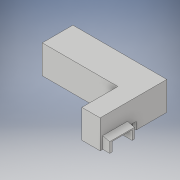
# Autodesk Inventor part: Батарейка
Saved by Autodesk Inventor 2019 (Build 230136000, 136)
## iProperties
Created: 2018-06-26
Part Number: Батарейка
Material: Типовые
Document SubType Name: Modeling
Designer: rossolov
Density: 1 g/cm^3
Appearance: По умолчанию
Author: rossolov
Autodesk Inventor part; units mm, degrees
ref_plane "YZ Plane" through (0, 0, 0) normal (1, 0, 0) x (0, 1, 0)
ref_plane "XZ Plane" through (0, 0, 0) normal (0, 1, 0) x (-1, 0, 0)
ref_plane "XY Plane" through (0, 0, 0) normal (0, 0, 1) x (1, 0, 0)
sketch "Эскиз1" plane through (0, 0, 0) normal (0, 0, 1) x (1, 0, 0)
  line L0 (-41.9106, 11.3854) -> (9.5324, 11.3854)
  line L1 (9.5324, 11.3854) -> (9.5324, -4.2346)
  line L2 (9.5324, -4.2346) -> (-41.9106, -4.2346)
  line L3 (-41.9106, -4.2346) -> (-41.9106, 11.3854)
  point P0 (0, 0)
  dimension "d0" = 51.443
  dimension "d1" = 15.62
  constraints: 8 end point, 2 parallel, 1 horizontal, 1 perpendicular
  measures "d0" distance of L1.end L2.end
  measures "d1" distance of L0.end L1.end
extrude "Выдавливание1" add sketch "Эскиз1" against normal blind 16.769
sketch "Эскиз2" plane through (9.5324, -4.2346, 0) normal (1, 0, 0) x (0, 0, -1)
  line L0 (0, 15.62) -> (16.769, 15.62) projected
  line L1 (16.769, 15.62) -> (-19.74, 15.62)
  line L2 (-19.74, 15.62) -> (-19.74, 0)
  line L3 (-19.74, 0) -> (16.769, 0)
  line L4 (16.769, 0) -> (16.769, 15.62)
  point P0 (0, 4.2346)
  dimension "d4" = 36.509
  constraints: 8 end point, 2 parallel, 1 horizontal, 1 perpendicular
  measures "d4" distance of L3.end L2.end
extrude "Выдавливание2" add sketch "Эскиз2" against normal blind 10
sketch "Эскиз3" plane through (9.5324, -4.2346, -16.769) normal (1, 0, 0) x (0, 0, -1)
  line L0 (0, 15.62) -> (0, 0) projected
  line L1 (-36.509, 0) -> (0, 0) projected
  line L2 (-16.769, 0) -> (-21.568, 0)
  line L3 (-21.568, 0) -> (-21.568, 4.078)
  line L4 (-21.568, 4.078) -> (-16.769, 4.078)
  line L5 (-16.769, 4.078) -> (-16.769, 0)
  point P0 (-16.769, 4.2346)
  dimension "d7" = 16.769
  dimension "d8" = 4.799
  dimension "d9" = 4.078
  constraints: 8 end point, 2 parallel, 1 horizontal, 1 perpendicular, 1 point on line
  measures "d7" distance of L0.end L2.start
  measures "d8" distance of L3.end L4.end
  measures "d9" distance of L2.end L3.end
extrude "Выдавливание3" cut sketch "Эскиз3" against normal blind 1.867
sketch "Эскиз4" plane through (-0.4676, -4.2346, 0) normal (-1, 0, 0) x (0, 0, 1)
  line L0 (19.74, 15.62) -> (19.74, 0) projected
  line L1 (18.24, 1.5) -> (1.5, 1.5)
  line L2 (1.5, 1.5) -> (1.5, 14.12)
  line L3 (1.5, 14.12) -> (18.24, 14.12)
  line L4 (18.24, 14.12) -> (18.24, 1.5)
  point P0 (0, 4.2346)
  constraints: 8 end point, 2 parallel, 1 horizontal, 1 perpendicular
extrude "Выдавливание4" cut sketch "Эскиз4" against normal blind 7.5
sketch "Эскиз6" plane through (9.5324, -4.2346, -16.769) normal (1, 0, 0) x (0, 0, -1)
  line L0 (-16.769, 0) -> (-36.509, 0) projected
  line L1 (-21.817, 0) -> (-22.817, 0)
  line L2 (-33.817, 5) -> (-22.817, 5)
  line L3 (-28.317, 6.7654) -> (-28.317, -1.5681)
  line L4 (-36.509, 0) -> (-21.568, 0) projected
  line L5 (-33.817, 5) -> (-33.817, 0)
  line L6 (-22.817, 5) -> (-22.817, 0)
  line L7 (-35.1049, 6.5) -> (-35.1049, 0)
  line L8 (-35.1049, 0) -> (-33.817, 0)
  line L9 (-35.1049, 6.5) -> (-21.568, 6.5)
  line L10 (-21.568, 6.5) -> (-21.568, 0)
  line L11 (-21.568, 0) -> (-21.568, 4.078) projected
  line L12 (-21.568, 0) -> (-22.817, 0)
  point P0 (-16.769, 4.2346)
  dimension "d20" = 1
  dimension "d27" = 5
  constraints: 20 end point, 4 point on line, 2 collinear, 2 perpendicular, 2 vertical, 1 horizontal, 1 parallel
  measures "d20" distance of L1.start L1.end
  measures "d27" distance between parallel lines of L0 L2
extrude "Выдавливание6" add sketch "Эскиз6" along normal blind 3.817 contours L0 L6 L2 L3 L9 L10 | L3 L2 L5 L0 L7 L9
sketch "Эскиз7" plane through (9.5324, -0.1566, 4.799) normal (0, 0, -1) x (-1, 0, 0)
  line L0 (-3.817, 1.491) -> (0, 2.422)
  line L1 (0, 11.542) -> (0, -4.078) projected
  line L2 (0, 2.422) -> (-3.817, 2.422) projected
  line L3 (0, 2.422) -> (-3.817, 2.422)
  line L4 (-3.817, 2.422) -> (-3.817, 1.491)
  point P0 (9.5324, 0.1566)
  point P1 (-3.817, -4.078)
  constraints: 6 end point, 1 collinear, 1 perpendicular, 1 point on line
extrude "Выдавливание7" cut sketch "Эскиз7" against normal blind 13.54
sketch "Эскиз8" plane through (-41.9106, -4.2346, -16.769) normal (0, -1, 0) x (1, 0, 0)
  line L0 (51.443, 33.817) -> (55.26, 33.817) projected
  line L1 (55.26, 33.817) -> (50.26, 33.817)
  line L2 (55.26, 33.817) -> (55.26, 22.817) projected
  line L3 (55.26, 22.817) -> (50.26, 22.817)
  line L4 (50.26, 22.817) -> (50.26, 33.817)
  line L5 (55.26, 22.817) -> (55.26, 33.817)
  point P0 (41.9106, 16.769)
  dimension "d33" = 5
  dimension "d34" = 5
  constraints: 8 end point, 1 collinear, 1 horizontal
  measures "d33" distance of L0.end L1.end
  measures "d34" distance of L2.end L3.end
extrude "Выдавливание8" cut sketch "Эскиз8" against normal blind 5
sketch "Эскиз10" plane through (8.3494, -4.2346, 17.048) normal (1, 0, 0) x (0, 0, -1)
  line L0 (0, 0) -> (0, 5) projected
  line L1 (0, 5) -> (0, 1)
  line L2 (0, 1) -> (11, 1)
  line L3 (11, 5) -> (11, 0) projected
  line L4 (11, 1) -> (11, 5)
  line L5 (0, 5) -> (11, 5) projected
  line L6 (11, 5) -> (0, 5)
  point P0 (17.048, 4.2346)
  dimension "d38" = 4
  constraints: 8 end point, 2 point on line, 1 collinear, 1 perpendicular, 1 vertical
  measures "d38" distance of L0.end L1.end
extrude "Выдавливание9" cut sketch "Эскиз10" against normal blind 10
sketch "Эскиз11" plane through (-0.4676, -4.2346, 0) normal (-1, 0, 0) x (0, 0, 1)
  line L0 (17.048, 0) -> (17.048, 5) projected
  line L1 (18.3359, 5.569) -> (18.3359, 0) projected
  line L2 (18.3359, 0.9988) -> (18.3359, 14.12)
  line L3 (1.5, 14.12) -> (18.24, 14.12) projected
  line L4 (18.3359, 14.12) -> (1.5, 14.12)
  line L5 (1.5, 14.12) -> (1.5, 0.9988)
  line L6 (1.5, 1.5) -> (1.5, 14.12) projected
  line L7 (1.5, 0.9988) -> (18.3359, 0.9988)
  point P0 (0, 4.2346)
  constraints: 8 end point, 3 collinear, 1 point on line
extrude "Выдавливание10" cut sketch "Эскиз11" against normal blind 7.817
